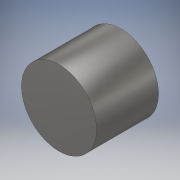
# Autodesk Inventor part: motor
Saved by Autodesk Inventor 2019 (Build 230136000, 136)
## iProperties
Created: 2019-04-07
Part Number: motor
Material: Stainless Steel
Document SubType Name: Modeling
Designer: albaa
Mass: 249.749 g
Surface Area: 55.1186 cm^2
Volume: 31.2186 cm^3
Density: 8 g/cm^3
Appearance: Semi-Polished
Author: albaa
Autodesk Inventor part; units mm, degrees
ref_plane "YZ Plane" through (0, 0, 0) normal (1, 0, 0) x (0, 1, 0)
ref_plane "XZ Plane" through (0, 0, 0) normal (0, 1, 0) x (-1, 0, 0)
ref_plane "XY Plane" through (0, 0, 0) normal (0, 0, 1) x (1, 0, 0)
sketch "Sketch2" plane through (0, 0, 0) normal (0, 0, 1) x (1, 0, 0)
  circle A0 centre (0, 0) radius 18.2
  dimension "d0" = 36.4
  constraints: 1 centre point, 1 coincident
  measures "d0" diameter of A0
extrude "Extrusion1" add sketch "Sketch2" along normal blind 15 and the other way blind 15
body "Solid1"
